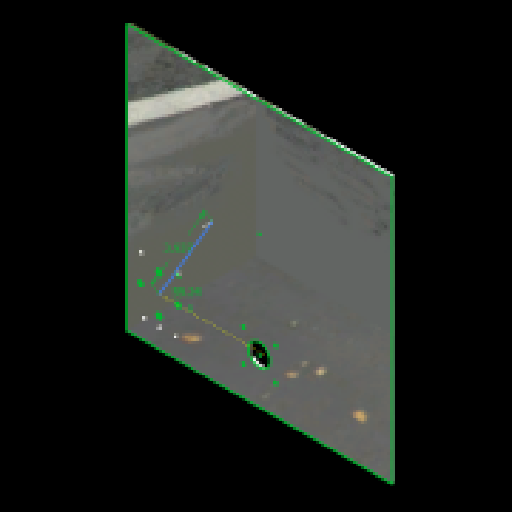
# Autodesk Inventor part: LeftAlPanel
Saved by Autodesk Inventor 2025 (Build 290162000, 162)
## iProperties
Created: 2025-01-19
Part Number: LeftAlPanel
Material: Aluminum 6061
Document SubType Name: Modeling
Designer: Trevor
Density: 2.7 g/cm^3
Appearance: Aluminum - Flat
Author: Trevor
Autodesk Inventor part; units mm, degrees
ref_plane "YZ Plane" through (0, 0, 0) normal (1, 0, 0) x (0, 1, 0)
ref_plane "XZ Plane" through (0, 0, 0) normal (0, 1, 0) x (-1, 0, 0)
ref_plane "XY Plane" through (0, 0, 0) normal (0, 0, 1) x (1, 0, 0)
sketch "Sketch1" plane through (0, 0, 0) normal (0, 0, 1) x (1, 0, 0)
  line L0 (0, 110.6854) -> (-127, 110.6854)
  line L1 (-127, 110.6854) -> (-127, -143.3146)
  line L2 (-127, -143.3146) -> (0, -143.3146)
  line L3 (-127, 110.6854) -> (127, 110.6854) projected
  line L4 (-127, -143.3146) -> (-127, 110.6854) projected
  line L5 (127, -143.3146) -> (-127, -143.3146) projected
  line L6 (127, 110.6854) -> (127, -143.3146) projected
  line L7 (0, 110.6854) -> (127, 110.6854)
  line L8 (127, 110.6854) -> (127, -143.3146)
  line L9 (127, -143.3146) -> (0, -143.3146)
  circle A0 centre (15.4948, -84.6086) radius 1.3281 projected
  circle A1 centre (0, -100.1034) radius 10.5 projected
  circle A2 centre (-15.4948, -115.5982) radius 1.3281 projected
  circle A3 centre (-15.4948, -84.6086) radius 1.3281 projected
  circle A4 centre (15.4948, -115.5982) radius 1.3281 projected
  circle A5 centre (-113.85, -97.5687) radius 2.5 projected
  circle A6 centre (-77.85, -97.5687) radius 2.5 projected
  circle A7 centre (-95.85, -79.5687) radius 2.5 projected
  circle A8 centre (-95.85, -115.5687) radius 2.5 projected
  point P0 (0, 0)
  point P1 (29.6393, -143.3146)
  point P2 (-29.6393, -143.3146)
  dimension "d0" = 254
  dimension "d1" = 127
  constraints: 12 end point, 2 parallel, 1 horizontal, 1 perpendicular, 2 other
  measures "d0" distance of L2.end L0.start
  measures "d1" distance of L0.end L0.start
extrude "Extrusion1" add sketch "Sketch1" along normal blind 3.175 contours L3 L6 L5 L2 L1 L0 | A0 | A1 | A2 | A3 | A4 | A5 | A6 | A7 | A8
sketch "Sketch3" plane through (0, 0, 0) normal (0, 0, -1) x (-1, 0, 0)
  circle A0 centre (0, -100.1034) radius 10.5
  spline S0 degree 2 number of poles 163
  spline S1 degree 2 number of poles 163
  spline S2 degree 2 number of poles 163
  spline S3 degree 2 number of poles 163
  circle A1 centre (-15.4948, -84.6086) radius 1.3281
  circle A2 centre (15.4948, -84.6086) radius 1.3281
  circle A3 centre (15.4948, -115.5982) radius 1.3281
  circle A4 centre (-15.4948, -115.5982) radius 1.3281
  point P0 (0, 0)
  point P1 (-15.4948, -83.0805)
  point P2 (-16.4994, -85.7601)
  constraints: 1 centre point, 1 horizontal alignment, 1 vertical alignment, 10 other
extrude "Extrusion3" cut sketch "Sketch3" against normal up to surface (3.175 mm away)
sketch "Sketch4" plane through (0, 0, 0) normal (0, 0, -1) x (-1, 0, 0)
  circle A0 centre (110.85, -124.0687) radius 2.5 projected
  circle A1 centre (78.1, -71.0687) radius 2.5 projected
  circle A2 centre (113.5793, -71.0687) radius 2.5 projected
  circle A3 centre (110.85, -124.0687) radius 2.5 projected
  circle A4 centre (95.85, -124.0687) radius 2.5 projected
  circle A5 centre (80.85, -124.0687) radius 2.5 projected
  line L0 (117.35, -68.0687) -> (117.35, -127.0687) projected
  line L1 (111.8085, -66.0687) -> (115.35, -66.0687) projected
  line L2 (109.8085, -68.0687) -> (109.8085, -76.5687) projected
  line L3 (109.8085, -76.5687) -> (112.4358, -76.5687) projected
  arc A6 (113.1429, -76.8616) -> (112.4358, -76.5687) centre (112.4358, -77.5687) ccw projected
  line L4 (113.1429, -76.8616) -> (116.5571, -80.2758) projected
  arc A7 (116.85, -80.9829) -> (116.5571, -80.2758) centre (115.85, -80.9829) ccw projected
  line L5 (116.85, -80.9829) -> (116.85, -83.3972) projected
  line L6 (116.85, -83.3972) -> (116.4142, -82.9614) projected
  arc A8 (117, -84.3756) -> (116.4142, -82.9614) centre (115, -84.3756) ccw projected
  line L7 (117, -84.3756) -> (117, -110.7619) projected
  arc A9 (116.4142, -112.1761) -> (117, -110.7619) centre (115, -110.7619) ccw projected
  line L8 (116.4142, -112.1761) -> (116.85, -111.7403) projected
  line L9 (116.85, -111.7403) -> (116.85, -114.1545) projected
  arc A10 (116.5571, -114.8616) -> (116.85, -114.1545) centre (115.85, -114.1545) ccw projected
  line L10 (116.5571, -114.8616) -> (113.1429, -118.2758) projected
  arc A11 (112.4358, -118.5687) -> (113.1429, -118.2758) centre (112.4358, -117.5687) ccw projected
  line L11 (112.4358, -118.5687) -> (110.0216, -118.5687) projected
  line L12 (110.0216, -118.5687) -> (110.4574, -118.1329) projected
  arc A12 (109.0431, -118.7187) -> (110.4574, -118.1329) centre (109.0431, -116.7187) ccw projected
  line L13 (109.0431, -118.7187) -> (82.6569, -118.7187) projected
  arc A13 (81.8969, -118.5687) -> (82.6569, -118.7187) centre (82.6569, -116.7187) ccw projected
  line L14 (81.8969, -118.5687) -> (79.2642, -118.5687) projected
  arc A14 (78.5571, -118.2758) -> (79.2642, -118.5687) centre (79.2642, -117.5687) ccw projected
  line L15 (78.5571, -118.2758) -> (75.1429, -114.8616) projected
  arc A15 (74.85, -114.1545) -> (75.1429, -114.8616) centre (75.85, -114.1545) ccw projected
  line L16 (74.85, -114.1545) -> (74.85, -111.5218) projected
  arc A16 (74.7, -110.7619) -> (74.85, -111.5218) centre (76.7, -110.7619) ccw projected
  line L17 (74.7, -110.7619) -> (74.7, -84.3756) projected
  arc A17 (74.85, -83.6157) -> (74.7, -84.3756) centre (76.7, -84.3756) ccw projected
  line L18 (74.85, -83.6157) -> (74.85, -80.9829) projected
  arc A18 (75.1429, -80.2758) -> (74.85, -80.9829) centre (75.85, -80.9829) ccw projected
  line L19 (75.1429, -80.2758) -> (78.5571, -76.8616) projected
  arc A19 (79.2642, -76.5687) -> (78.5571, -76.8616) centre (79.2642, -77.5687) ccw projected
  line L20 (79.2642, -76.5687) -> (81.8915, -76.5687) projected
  line L21 (81.8915, -76.5687) -> (81.8915, -76.0687) projected
  line L22 (81.8915, -76.0687) -> (81.85, -76.0687) projected
  line L23 (81.85, -68.0687) -> (81.85, -76.0687) projected
  line L24 (76.35, -66.0687) -> (79.85, -66.0687) projected
  line L25 (74.35, -127.0687) -> (74.35, -68.0687) projected
  line L26 (115.35, -129.0687) -> (76.35, -129.0687) projected
  circle A20 centre (80.85, -124.0687) radius 2.5 projected
  circle A21 centre (113.5793, -71.0687) radius 2.5 projected
  circle A22 centre (78.1, -71.0687) radius 2.5 projected
  arc A23 (115.35, -129.0687) -> (117.35, -127.0687) centre (115.35, -127.0687) ccw projected
  arc A24 (117.35, -68.0687) -> (115.35, -66.0687) centre (115.35, -68.0687) ccw projected
  arc A25 (111.8085, -66.0687) -> (109.8085, -68.0687) centre (111.8085, -68.0687) ccw projected
  arc A26 (81.85, -68.0687) -> (79.85, -66.0687) centre (79.85, -68.0687) ccw projected
  arc A27 (76.35, -66.0687) -> (74.35, -68.0687) centre (76.35, -68.0687) ccw projected
  arc A28 (74.35, -127.0687) -> (76.35, -129.0687) centre (76.35, -127.0687) ccw projected
  point P0 (0, 0)
extrude "Extrusion4" cut sketch "Sketch4" against normal up to surface (3.175 mm away) contours A0 | A1 | A2 | A4 | A5
sketch "Sketch5" plane through (0, 0, 3.175) normal (0, 0, 1) x (1, 0, 0)
  circle A0 centre (-113.85, -97.5687) radius 2.5 projected
  circle A1 centre (-77.85, -97.5687) radius 2.5 projected
  circle A2 centre (-95.85, -79.5687) radius 2.5 projected
  circle A3 centre (-95.85, -115.5687) radius 2.5 projected
  circle A4 centre (15.4948, -84.6086) radius 1.3281 projected
  circle A5 centre (0, -100.1034) radius 10.5 projected
  circle A6 centre (-15.4948, -115.5982) radius 1.3281 projected
  circle A7 centre (-15.4948, -84.6086) radius 1.3281 projected
  circle A8 centre (15.4948, -115.5982) radius 1.3281 projected
  line L0 (-127, 110.6854) -> (127, 110.6854) projected
  line L1 (-127, -143.3146) -> (-127, 110.6854) projected
  line L2 (127, -143.3146) -> (-127, -143.3146) projected
  line L3 (127, 110.6854) -> (127, -143.3146) projected
  circle A9 centre (-113.85, -97.5687) radius 2.5 projected
  circle A10 centre (-77.85, -97.5687) radius 2.5 projected
  circle A11 centre (-95.85, -79.5687) radius 2.5 projected
  circle A12 centre (-95.85, -115.5687) radius 2.5 projected
  circle A13 centre (15.4948, -84.6086) radius 1.3281 projected
  circle A14 centre (0, -100.1034) radius 10.5 projected
  circle A15 centre (-15.4948, -115.5982) radius 1.3281 projected
  circle A16 centre (-15.4948, -84.6086) radius 1.3281 projected
  circle A17 centre (15.4948, -115.5982) radius 1.3281 projected
  line L4 (-127, 110.6854) -> (127, 110.6854) projected
  line L5 (-127, -143.3146) -> (-127, 110.6854) projected
  line L6 (127, -143.3146) -> (-127, -143.3146) projected
  line L7 (127, 110.6854) -> (127, -143.3146) projected
  circle A18 centre (-113.85, -97.5687) radius 2.5 projected
  circle A19 centre (-77.85, -97.5687) radius 2.5 projected
  circle A20 centre (-95.85, -79.5687) radius 2.5 projected
  circle A21 centre (-95.85, -115.5687) radius 2.5 projected
  circle A22 centre (15.4948, -84.6086) radius 1.3281 projected
  circle A23 centre (0, -100.1034) radius 10.5 projected
  circle A24 centre (-15.4948, -115.5982) radius 1.3281 projected
  circle A25 centre (-15.4948, -84.6086) radius 1.3281 projected
  circle A26 centre (15.4948, -115.5982) radius 1.3281 projected
  line L8 (-127, 110.6854) -> (127, 110.6854) projected
  line L9 (-127, -143.3146) -> (-127, 110.6854) projected
  line L10 (127, -143.3146) -> (-127, -143.3146) projected
  line L11 (127, 110.6854) -> (127, -143.3146) projected
  circle A27 centre (-113.85, -97.5687) radius 2.5 projected
  circle A28 centre (-77.85, -97.5687) radius 2.5 projected
  circle A29 centre (-95.85, -79.5687) radius 2.5 projected
  circle A30 centre (-95.85, -115.5687) radius 2.5 projected
  circle A31 centre (15.4948, -84.6086) radius 1.3281 projected
  circle A32 centre (0, -100.1034) radius 10.5 projected
  circle A33 centre (-15.4948, -115.5982) radius 1.3281 projected
  circle A34 centre (-15.4948, -84.6086) radius 1.3281 projected
  circle A35 centre (15.4948, -115.5982) radius 1.3281 projected
  line L12 (-127, 110.6854) -> (127, 110.6854) projected
  line L13 (-127, -143.3146) -> (-127, 110.6854) projected
  line L14 (127, -143.3146) -> (-127, -143.3146) projected
  line L15 (127, 110.6854) -> (127, -143.3146) projected
  circle A36 centre (-113.85, -97.5687) radius 2.5 projected
  circle A37 centre (-77.85, -97.5687) radius 2.5 projected
  circle A38 centre (-95.85, -79.5687) radius 2.5 projected
  circle A39 centre (-95.85, -115.5687) radius 2.5 projected
  circle A40 centre (15.4948, -84.6086) radius 1.3281 projected
  circle A41 centre (0, -100.1034) radius 10.5 projected
  circle A42 centre (-15.4948, -115.5982) radius 1.3281 projected
  circle A43 centre (-15.4948, -84.6086) radius 1.3281 projected
  circle A44 centre (15.4948, -115.5982) radius 1.3281 projected
  line L16 (-127, 110.6854) -> (127, 110.6854) projected
  line L17 (-127, -143.3146) -> (-127, 110.6854) projected
  line L18 (127, -143.3146) -> (-127, -143.3146) projected
  line L19 (127, 110.6854) -> (127, -143.3146) projected
  line L20 (-95.85, -97.5687) -> (-44.7057, -11.637)
  line L21 (-95.85, -97.5687) -> (4.15, -97.5687) construction
  point P0 (0, 0)
  dimension "d11" = 100
  dimension "d12" = 59.24
  constraints: 4 end point, 1 equal length, 1 horizontal
  measures "d11" distance of L20.start L20.end
  measures "d12" angle of L21 L20
body "Solid1"
